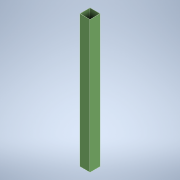
# Autodesk Inventor part: Pata_mesa
Saved by Autodesk Inventor 2021 (Build 250183000, 183)
## iProperties
Created: 2021-04-29
Part Number: Pata_mesa
Material: Genérico
Document SubType Name: Modeling
Designer: Admin
Density: 1 g/cm^3
Appearance: Default(1)
Author: Admin
Autodesk Inventor part; units mm, degrees
ref_plane "YZ Plane" through (0, 0, 0) normal (1, 0, 0) x (0, 1, 0)
ref_plane "XZ Plane" through (0, 0, 0) normal (0, 1, 0) x (-1, 0, 0)
ref_plane "XY Plane" through (0, 0, 0) normal (0, 0, 1) x (1, 0, 0)
sketch "Boceto1" plane through (0, 0, 0) normal (0, 1, 0) x (-1, 0, 0)
  line L0 (0, 0) -> (80, 0)
  line L1 (80, 0) -> (80, -80)
  line L2 (80, -80) -> (0, -80)
  line L3 (0, -80) -> (0, 0)
  line L4 (1.5, -78.5) -> (78.5, -78.5)
  line L5 (78.5, -78.5) -> (78.5, -1.5)
  line L6 (78.5, -1.5) -> (1.5, -1.5)
  line L7 (1.5, -1.5) -> (1.5, -78.5)
  line L8 (1.5, -78.5) -> (78.5, -1.5) construction
  line L9 (78.5, -78.5) -> (1.5, -1.5) construction
  point P0 (40, -40)
  dimension "d0" = 80
  dimension "d1" = 80
  dimension "d2" = 77
  dimension "d3" = 77
  constraints: 20 end point, 4 parallel, 2 horizontal, 2 midpoint, 2 perpendicular
  measures "d0" distance of L1.end L2.end
  measures "d1" distance of L0.end L1.end
  measures "d2" distance of L6.end L5.end
  measures "d3" distance of L5.end L4.end
extrude "Extrusión1" add sketch "Boceto1" along normal blind 1030.856
